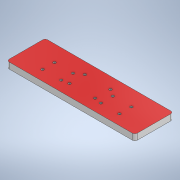
# Autodesk Inventor part: Placa Herramienta
Saved by Autodesk Inventor 2021 (Build 250183000, 183)
## iProperties
Created: 2022-01-21
Part Number: Placa Herramienta
Material: Generic
Document SubType Name: Modeling
Designer: deuts
Density: 1 g/cm^3
Appearance: Default
Author: deuts
Autodesk Inventor part; units mm, degrees
ref_plane "YZ Plane" through (0, 0, 0) normal (1, 0, 0) x (0, 1, 0)
ref_plane "XZ Plane" through (0, 0, 0) normal (0, 1, 0) x (-1, 0, 0)
ref_plane "XY Plane" through (0, 0, 0) normal (0, 0, 1) x (1, 0, 0)
sketch "Sketch1" plane through (0, 0, 0) normal (0, 1, 0) x (-1, 0, 0)
  line L0 (-100, 30) -> (100, 30)
  line L1 (100, 30) -> (100, -30)
  line L2 (100, -30) -> (-100, -30)
  line L3 (-100, -30) -> (-100, 30)
  circle A0 centre (60, 14) radius 2
  circle A1 centre (31, 14) radius 2
  circle A2 centre (-31, 14) radius 2
  circle A3 centre (-60, 14) radius 2
  circle A4 centre (20, 12) radius 2
  circle A5 centre (-20, 12) radius 2
  circle A6 centre (60, -4.55) radius 2
  circle A7 centre (31, -4.55) radius 2
  circle A8 centre (20, -12) radius 2
  circle A9 centre (-20, -12) radius 2
  circle A10 centre (-31, -4.55) radius 2
  circle A11 centre (-60, -4.55) radius 2
  point P0 (0, 0)
  dimension "d0" = 200
  dimension "d1" = 60
  dimension "d7" = 4
  dimension "d12" = 4
  dimension "d15" = 4
  dimension "d16" = 4
  dimension "d18" = 4
  dimension "d19" = 4
  dimension "d23" = 4
  dimension "d24" = 4
  dimension "d25" = 18.55
  dimension "d30" = 100
  constraints: 12 centre point, 8 end point, 2 parallel, 1 horizontal, 1 perpendicular
  measures "d0" distance of L1.end L2.end
  measures "d1" distance of L0.end L1.end
  measures "d7" diameter of A0
  measures "d12" diameter of A4
  measures "d15" diameter of A6
  measures "d16" diameter of A7
  measures "d18" diameter of A8
  measures "d19" diameter of A9
  measures "d23" diameter of A10
  measures "d24" diameter of A11
  measures "d25" distance of A2.centre A10.centre
  measures "d30" distance from line of point (0, 0) L1
extrude "Extrusion1" add sketch "Sketch1" along normal blind 9.525 contours L0 L1 L2 L3 | A10 | A11
fillet "Fillet1" radius 4 4 edges at (100, 4.7625, -30) (-100, 4.7625, -30) (100, 4.7625, 30) (-100, 4.7625, 30)
sketch "Sketch2" plane through (0, 9.525, 0) normal (0, 1, 0) x (1, 0, 0)
  circle A0 centre (31, -14) radius 2 projected
  circle A1 centre (60, -14) radius 2 projected
  circle A2 centre (31, 4.55) radius 2
  circle A3 centre (60, 4.55) radius 2
  point P0 (0, 0)
  dimension "d26" = 4
  dimension "d27" = 4
  constraints: 2 centre point
  measures "d26" diameter of A2
  measures "d27" diameter of A3
extrude "Extrusion2" cut sketch "Sketch2" against normal blind 9.525 contours A2 | A3
body "Solid1"
